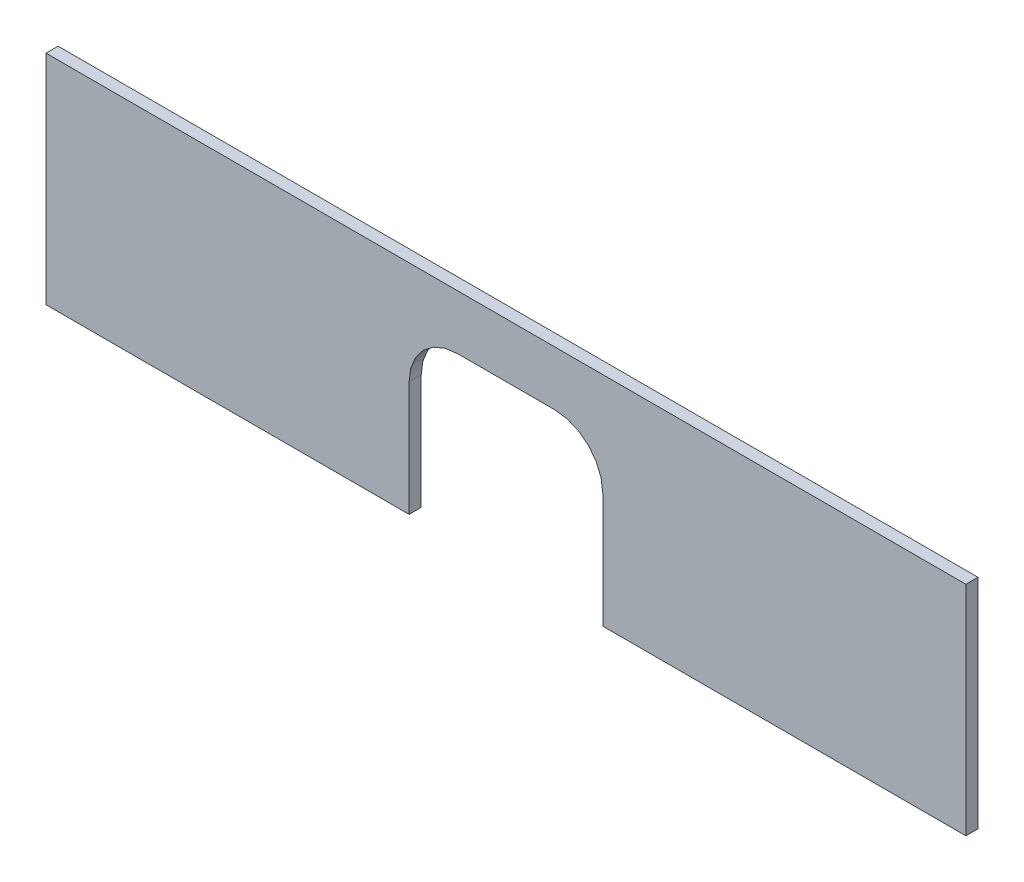
# Autodesk Inventor part: plywood front pannel
Saved by Autodesk Inventor 2012 (Build 160160000, 160)
## iProperties
Created: 2013-09-02
Part Number: plywood front pannel
Material: Default
Document SubType Name: Modeling
Designer: Bryce
Density: 1 g/cm^3
Author: Bryce
Autodesk Inventor part; units mm, degrees
ref_plane "YZ Plane" through (0, 0, 0) normal (1, 0, 0) x (0, 1, 0)
ref_plane "XZ Plane" through (0, 0, 0) normal (0, 1, 0) x (-1, 0, 0)
ref_plane "XY Plane" through (0, 0, 0) normal (0, 0, 1) x (1, 0, 0)
sketch "Sketch1" plane through (0, 0, 0) normal (0, 0, 1) x (1, 0, 0)
  line L0 (965.2, 0) -> (965.2, 228.6)
  line L1 (965.2, 228.6) -> (0, 228.6)
  line L2 (0, 228.6) -> (0, 0)
  line L3 (584.2, 0) -> (584.2, 120.65)
  line L4 (584.2, 171.45) -> (533.4, 171.45) construction
  line L5 (381, 171.45) -> (381, 120.65) construction
  line L6 (0, 0) -> (381, 0)
  line L7 (584.2, 0) -> (965.2, 0)
  arc A0 (431.8, 171.45) -> (381, 120.65) centre (431.8, 120.65) ccw
  arc A1 (584.2, 120.65) -> (533.4, 171.45) centre (533.4, 120.65) ccw
  line L8 (431.8, 171.45) -> (381, 171.45) construction
  line L9 (381, 120.65) -> (381, 0)
  line L10 (533.4, 171.45) -> (431.8, 171.45)
  line L11 (584.2, 120.65) -> (584.2, 171.45) construction
  dimension "d0" = 965.2
  dimension "d1" = 228.6
  dimension "d4" = 203.2
  dimension "d6" = 381
  dimension "d7" = 171.45
  dimension "d8" = 50.8
  constraints: 24 end point, 10 tangent, 8 perpendicular, 7 parallel, 4 point on circle, 2 centre point, 2 horizontal, 1 collinear, 1 equal radius
  measures "d0" distance of L0.end L1.end
  measures "d1" distance of L1.end L2.end
  measures "d4" distance of L4.start L5.start
  measures "d6" distance between parallel lines of L2 L5
  measures "d7" distance of L5.start L6.end
  measures "d8" radius of A0
extrude "Extrusion1" add sketch "Sketch1" along normal blind 12.7
equation "\"d6\" = 0.5 * d0 - 0.5 * d4"
body "Solid1"
